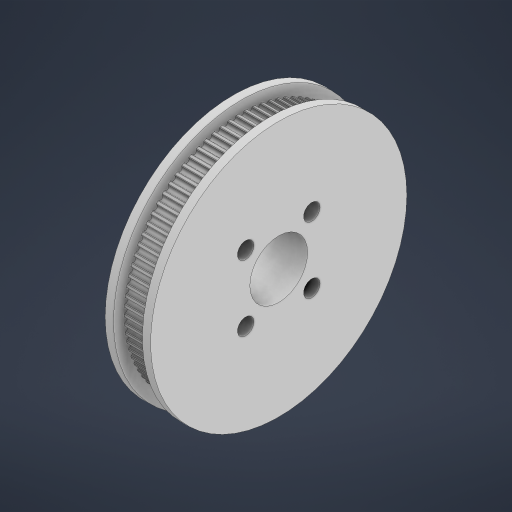
# Autodesk Inventor part: GT2 Pulley
Saved by Autodesk Inventor 2024 (Build 280153000, 153)
## iProperties
Created: 2023-10-25
Part Number: GT2 Pulley
Material: Generic
Document SubType Name: Modeling
Designer: avsar
Density: 1 g/cm^3
Appearance: Default
Author: avsar
Autodesk Inventor part; units mm, degrees
ref_plane "YZ Plane" through (0, 0, 0) normal (1, 0, 0) x (0, 1, 0)
ref_plane "XZ Plane" through (0, 0, 0) normal (0, 1, 0) x (-1, 0, 0)
ref_plane "XY Plane" through (0, 0, 0) normal (0, 0, 1) x (1, 0, 0)
sketch "Sketch1" plane through (0, 0, 0) normal (1, 0, 0) x (0, 1, 0)
  circle A0 centre (0, 0) radius 28.3939 construction
  circle A1 centre (0, 0) radius 27.6439 construction
  line L0 (0, 0) -> (28.3939, 0) construction
  line L1 (0, 0) -> (0, -28.3939) construction
  circle A2 centre (28.1989, 0) radius 0.555 construction
  line L2 (0, 0) -> (28.3247, -1.9807) construction
  circle A3 centre (28.1302, -1.9671) radius 0.555 construction
  circle A4 centre (28.2351, -0.7041) radius 0.15 construction
  circle A5 centre (28.2154, -1.2672) radius 0.15 construction
  arc A6 (27.6439, 0) -> (28.2274, -0.5543) centre (28.1989, 0) ccw
  arc A7 (28.3851, -0.7078) -> (28.2274, -0.5543) centre (28.2351, -0.7041) ccw
  arc A8 (28.3653, -1.274) -> (28.3851, -0.7078) centre (0, 0) ccw
  arc A9 (28.1973, -1.4161) -> (28.3653, -1.274) centre (28.2154, -1.2672) ccw
  arc A10 (28.1973, -1.4161) -> (27.5766, -1.9283) centre (28.1302, -1.9671) ccw
  arc A11 (27.5766, -1.9283) -> (27.6439, 0) centre (0, 0) ccw
  dimension "d0" = 56.7878
  dimension "d1" = -0.75
  dimension "d2" = 1.11
  dimension "d4" = 86
  dimension "d5" = 0.3
  constraints: 25 point on circle, 12 centre point, 8 equal radius, 8 tangent, 6 end point, 4 point on line, 1 coincident, 1 concentric, 1 horizontal, 1 perpendicular
  measures "d0" diameter of A0
  measures "d1" radial gap between concentric circles of A0 A1
  measures "d2" diameter of A2
  measures "d4" angle of L1 L2
  measures "d5" diameter of A4
extrude "Extrusion1" add sketch "Sketch1" along normal mid plane 7
pattern_circular "Circular Pattern1" count 90 over 360 about axis through (-10, 0, 0) along (1, 0, 0) of "Extrusion1"
sketch "Sketch2" plane through (0, 0, 0) normal (1, 0, 0) x (0, 1, 0)
  arc A0 (27.5766, 1.9283) -> (28.1973, 1.4161) centre (28.1302, 1.9671) ccw projected
  circle A1 centre (0, 0) radius 27.6439
  constraints: 1 coincident, 3 other
extrude "Extrusion2" add sketch "Sketch2" along normal mid plane 7
sketch "Sketch3" plane through (3.5, 0, 0) normal (1, 0, 0) x (0, 0, -1)
  circle A0 centre (0, 0) radius 31
  dimension "d13" = 62
  constraints: 1 centre point, 1 coincident
  measures "d13" diameter of A0
extrude "Extrusion3" add sketch "Sketch3" along normal blind 2
sketch "Sketch4" plane through (-3.5, 0, 0) normal (-1, 0, 0) x (0, 0, 1)
  circle A0 centre (0, 0) radius 31 projected
extrude "Extrusion4" add sketch "Sketch4" along normal blind 2
sketch "Sketch5" plane through (5.5, 0, 0) normal (1, 0, 0) x (0, 0, -1)
  circle A0 centre (0, 0) radius 7
  circle A1 centre (-8, 8) radius 2
  circle A2 centre (-8, -8) radius 2
  circle A3 centre (8, -8) radius 2
  circle A4 centre (8, 8) radius 2
  dimension "d18" = 14
  dimension "d19" = 4
  dimension "d20" = 8
  dimension "d21" = 8
  dimension "d24" = 360
  constraints: 5 centre point, 1 coincident, 9 other
  measures "d18" diameter of A0
  measures "d19" diameter of A1
  measures "d20" horizontal distance of point (0, 0) A1.centre
  measures "d21" horizontal distance of point (0, 0) A1.centre
extrude "Extrusion5" cut sketch "Sketch5" against normal through all
equation "\"d0\" = OD_"
equation "\"d1\" = H_"
equation "\"d2\" = BTD_"
equation "\"d4\" = TH_"
equation "\"d5\" = PTR_"
equation "\"d6\" = EX_"
equation "\"d11\" = EX_"
equation "\"U_\" = 0.254"
equation "\"H_\" = -0.75"
equation "\"P_\" = 2"
equation "\"BTD_\" = 1.11"
equation "\"PTR_\" = 0.3"
equation "\"EX_\" = 7"
equation "\"OD_\" = PD_ - 2 * U_"
equation "\"TH_\" = 86deg"
equation "\"PD_\" = 57.29578"
body "Solid1"
